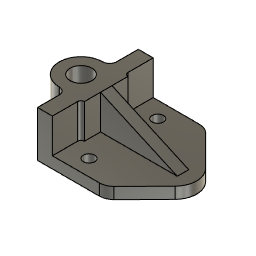
A3 (Autodesk Fusion 360 design; units mm, degrees)
Autodesk Fusion 360 part; units mm, degrees
sketch "Sketch1" plane through (0, 0, 0) normal (0, 0, 1) x (1, 0, 0)
  line L0 (0, 50) -> (53.404, 50)
  line L1 (54, -38) -> (0, -38)
  line L2 (0, -38) -> (0, 50)
  arc A0 (54, -38) -> (63.0412, -34.3412) centre (54, -25) ccw
  arc A1 (62.6413, 46.1473) -> (53.404, 50) centre (53.404, 37) ccw
  line L3 (63.0412, -34.3412) -> (89.552, -7.4343)
  line L4 (89.4528, 19.3358) -> (62.6413, 46.1473)
  arc A2 (89.552, -7.4343) -> (89.4528, 19.3358) centre (76.0178, 5.9008) ccw
  circle A3 centre (31, -24) radius 5
  circle A4 centre (31, 36) radius 5
  dimension "d2" = 88
  dimension "d6" = 13
  dimension "d7" = 13
  dimension "d10" = 19
  dimension "d13" = 10
  dimension "d15" = 10
  constraint horizontal L0
  constraint horizontal L1
  constraint vertical L2
  constraint tangent L1 A0
  constraint tangent L0 A1
  constraint tangent L3 A2
  constraint tangent L4 A2
  measures "d2" distance of L0.start L1.end
  measures "d6" radius of A0
  measures "d7" radius of A1
  measures "d10" radius of A2
  measures "d13" diameter of A3
  measures "d15" diameter of A4
extrude "Extrude1" add sketch "Sketch1" along normal blind 10 makes body 1
sketch "Sketch2" plane through (0, 0, 10) normal (0, 0, 1) x (-1, 0, 0)
  circle A0 centre (-31, -36) radius 5
  circle A1 centre (-31, 24) radius 5
  arc A2 (-54, 38) -> (-63.0412, 34.3412) centre (-54, 25) ccw
  line L0 (-63.0412, 34.3412) -> (-89.552, 7.4343)
  arc A3 (-89.552, 7.4343) -> (-89.4528, -19.3358) centre (-76.0178, -5.9008) ccw
  line L1 (-89.4528, -19.3358) -> (-62.6413, -46.1473)
  arc A4 (-62.6413, -46.1473) -> (-53.404, -50) centre (-53.404, -37) ccw
  line L2 (-53.404, -50) -> (0, -50)
  line L3 (0, -50) -> (0, 38)
  line L4 (0, 38) -> (-54, 38)
  line L5 (0, 38) -> (-13, 38)
  line L6 (-13, 38) -> (-13, 16)
  line L7 (0, 13) -> (0, 38)
  line L8 (0, -50) -> (-13, -50)
  line L9 (-13, -50) -> (-13, -28)
  line L10 (0, -25) -> (0, -50)
  line L11 (-13, -25) -> (-16, -25)
  line L12 (-16, -25) -> (-16, -25)
  line L13 (25, -25) -> (25, 13)
  line L14 (-16, 13) -> (-16, 13)
  line L15 (-16, 13) -> (-16, -25)
  arc A5 (-16, 13) -> (-13, 16) centre (-16, 16) ccw
  arc A6 (-13, -28) -> (-16, -25) centre (-16, -28) ccw
  line L16 (25, 13) -> (6, 13)
  line L17 (25, -25) -> (0, -25)
  line L18 (0, -50) -> (0, -31)
  line L19 (6, -25) -> (25, -25)
  line L20 (25, -25) -> (25, 13)
  line L21 (25, 13) -> (0, 13)
  line L22 (0, 19) -> (0, 38)
  arc A7 (0, 19) -> (6, 13) centre (6, 19) ccw
  arc A8 (6, -25) -> (0, -31) centre (6, -31) ccw
  dimension "d18" = 13
  dimension "d19" = 25
  dimension "d20" = 13
  dimension "d21" = 25
  dimension "d23" = 41
  dimension "d24" = 3
  dimension "d25" = 3
  dimension "d26" = 6
  dimension "d27" = 6
  constraint horizontal L5
  constraint vertical L6
  constraint vertical L7
  constraint coincident L3.end L4.start
  constraint horizontal L8
  constraint vertical L9
  constraint vertical L10
  constraint coincident L2.end L3.start
  constraint perpendicular L9 L11
  constraint vertical L13
  constraint vertical L15
  constraint coincident L13.end L14
  constraint tangent L6 A5
  constraint coincident L13.start L12
  constraint coincident L11.start L9
  constraint tangent L9 A6
  constraint perpendicular L3 L17
  constraint parallel L13 L20
  constraint parallel L16 L21
  constraint coincident L7.start L22
  constraint tangent L16 A7
  constraint tangent L22 A7
  constraint coincident L10.start L19
  constraint coincident L10.start L18
  constraint tangent L19 A8
  constraint tangent L18 A8
  measures "d18" distance of L3.end L5.end
  measures "d19" distance of L3.end L7.start
  measures "d20" distance of L2.end L8.end
  measures "d21" distance of L2.end L10.start
  measures "d23" distance of L11.end L13.start
  measures "d24" radius of A5
  measures "d25" radius of A6
  measures "d26" radius of A7
  measures "d27" radius of A8
extrude "Extrude2" add sketch "Sketch2" against normal blind 10 contours L3 L7 L21 A7 | L3 L13 L16 L17 L19 L20 L21 | L3 L10 L17 A8 bodies 1
extrude "Extrude3" add sketch "Sketch2" along normal blind 30 contours L3 L7 L21 A7 | L3 L13 L16 L17 L19 L20 L21 | L3 L10 L17 A8 bodies 1
extrude "Extrude4" add sketch "Sketch2" along normal blind 30 contours L2 L3 L4 L5 L6 L7 L8 L9 L10 L15 A5 A6 L18 L22 bodies 1
fillet "Fillet1" radius 19 2 edges at (-25, -13, 20) (-25, 25, 20) on bodies 1
sketch "Sketch3" plane through (0, 0, 40) normal (0, 0, 1) x (-1, 0, 0)
  arc A0 (6, -25) -> (25, -6) centre (6, -6) ccw
  arc A1 (25, -6) -> (6, 13) centre (6, -6) ccw
  arc A2 (0, 19) -> (6, 13) centre (6, 19) ccw
  line L0 (0, 19) -> (0, 38)
  line L1 (0, 38) -> (-13, 38)
  line L2 (-13, 38) -> (-13, 16)
  arc A3 (-16, 13) -> (-13, 16) centre (-16, 16) ccw
  line L3 (-16, 13) -> (-16, -25)
  arc A4 (-13, -28) -> (-16, -25) centre (-16, -28) ccw
  line L4 (-13, -28) -> (-13, -50)
  line L5 (-13, -50) -> (0, -50)
  line L6 (0, -50) -> (0, -31)
  arc A5 (6, -25) -> (0, -31) centre (6, -31) ccw
  circle A6 centre (6, -6) radius 9.5
  dimension "d36" = 19
  constraint concentric A0 A6
  measures "d36" diameter of A6
extrude "Extrude5" cut sketch "Sketch3" against normal blind 40 contours A6 bodies 1
sketch "Sketch4" plane through (0, -38, 0) normal (0, -1, 0) x (1, 0, 0)
  line L0 (0, 0) -> (54, 0)
  line L1 (54, 0) -> (54, 10)
  line L2 (54, 10) -> (13, 10)
  line L3 (13, 10) -> (13, 40)
  line L4 (13, 40) -> (0, 40)
  line L5 (0, 40) -> (0, 0)
  line L6 (16.0173, 10) -> (83.0173, 10)
  line L7 (16.0173, 10) -> (16.0173, 40)
  line L8 (83.0173, 10) -> (16.0173, 40)
  dimension "d39" = 67
  dimension "d40" = 30
  constraint coincident L2 L6.start
  constraint perpendicular L3 L6
  constraint perpendicular L6 L7
  measures "d39" distance of L6.start L6.end
  measures "d40" distance of L6.start L7.end
extrude "Extrude6" add sketch "Sketch4" along normal blind 10 separate body contours L2 L6 L7 L8 makes body 2
move_body "Move1" bodies 2 to x (1, 0, 0) y (0, 1, 0) z (0, 0, 1) at (0, 49, 0)
combine "Combine1" operation add target body 1 tool bodies 2
named bodies: "A3"
